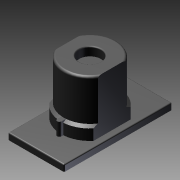
# Autodesk Inventor part: M2T12A5bush
Saved by Autodesk Inventor 2011 SP1 (Build 150282100, 282)
## iProperties
Created: 2013-12-24
Part Number: M2T12A5bush
Catalog Web Link: www.cadenas.de
Description: M2T Series - Process Sealed Miniature Toggles - Bushing-
Vendor: NKKSWITCHES
Document SubType Name: Modeling
Designer: PARTuser1
Manufacturer: NKKSWITCHES
Density: 1 g/cm^3
Category: PARTsolutions
Company: NKKSWITCHES
Title: M2T12A5bush
Author: Cadenas PARTsolutions
PSOL_IDENT_0: {$CADENAS_DATA\23d-libs\nkkswitches\toggle\m2t\parts\m2t_bushing.prj},222 {VTYP=3D},{NB=M2T12A5bush}
PSOL_IDENT_1: ,{LINA=M2T12A5bush},{NN=M2T Series - Process Sealed Miniature Toggles - Bushing},{DATE=07.04.2009 11
PSOL_IDENT_2: :51:13},{GEOMDATE=07.04.2009 11:51:00},{VERSION=},{LINEID=10},{LINESUBID=-1},{WBVAR=PLS,CRCTS}  {NB=
PSOL_IDENT_3: M2T12A5bush},{LINA=M2T12A5bush},{KT=DUMMY},{PN=M2T12A5},{SRS=M2T},{PLS=1},{CRCTS=2},{BSHNG=A5 - .250
PSOL_IDENT_4: \" (6.35mm) Double Flatted}
CNS_NN: M2T Series - Process Sealed Miniature Toggles - Bushing
CNS_NB: M2T12A5bush
CNS_NBSYN: $PN.bush
CNS_LINA: M2T12A5bush
CNS_PN: M2T12A5
CNS_SRS: M2T
CNS_PLS: 1 - SPDT
CNS_CRCTS: 2 - ON/NONE/ON
CNS_BSHNG: A5 - .250" (6.35mm) Double Flatted
SUPPLIER: NKKSWITCHES
ARTICLENO: M2T12A5bush
BOMINFO: M2T12A5bush
CREATOR: CADENAS GmbH
Autodesk Inventor part; units mm, degrees
sketch "Sketch_1" plane through (0, 0, 0) normal (0, 1, 0) x (-1, 0, 0)
  line L0 (3.302, -6.223) -> (3.302, 6.223)
  arc A0 (3.302, 6.223) -> (3.175, 6.35) centre (3.175, 6.223) ccw
  line L1 (3.175, 6.35) -> (-3.175, 6.35)
  arc A1 (-3.175, 6.35) -> (-3.302, 6.223) centre (-3.175, 6.223) ccw
  line L2 (-3.302, 6.223) -> (-3.302, -6.223)
  arc A2 (-3.302, -6.223) -> (-3.175, -6.35) centre (-3.175, -6.223) ccw
  line L3 (-3.175, -6.35) -> (3.175, -6.35)
  arc A3 (3.175, -6.35) -> (3.302, -6.223) centre (3.175, -6.223) ccw
  constraints: 8 end point, 8 point on circle, 4 centre point
extrude "Extrusion1" add sketch "Sketch_1" against normal blind 0.762
sketch "Sketch_2" plane through (0, 0, 0) normal (0, 0, 1) x (1, 0, 0)
  line L0 (-3.302, 0.254) -> (-3.302, -0.127)
  arc A0 (-3.175, 0) -> (-3.302, -0.127) centre (-3.175, -0.127) ccw
  line L1 (-3.175, 0) -> (3.175, 0)
  arc A1 (3.302, -0.127) -> (3.175, 0) centre (3.175, -0.127) ccw
  line L2 (3.302, -0.127) -> (3.302, 0.254)
  line L3 (3.302, 0.254) -> (-3.302, 0.254)
  constraints: 8 end point, 4 point on circle, 2 centre point
extrude "Extrusion2" cut sketch "Sketch_2" along normal mid plane 12.7
sketch "Sketch_3" plane through (0, 0, 0) normal (1, 0, 0) x (0, 1, 0)
  line L0 (0.254, 6.35) -> (-0.127, 6.35)
  arc A0 (0, 6.223) -> (-0.127, 6.35) centre (-0.127, 6.223) ccw
  line L1 (0, 6.223) -> (0, -6.223)
  arc A1 (-0.127, -6.35) -> (0, -6.223) centre (-0.127, -6.223) ccw
  line L2 (-0.127, -6.35) -> (0.254, -6.35)
  line L3 (0.254, -6.35) -> (0.254, 6.35)
  constraints: 8 end point, 4 point on circle, 2 centre point
extrude "Extrusion3" cut sketch "Sketch_3" along normal mid plane 12.7
sketch "Sketch_4" plane through (0, 0, 0) normal (1, 0, 0) x (0, 1, 0)
  line L0 (0, 0) -> (6.35, 0)
  line L1 (5.334, 0) -> (5.334, -1.27)
  line L2 (5.334, -1.27) -> (6.223, -1.27)
  arc A0 (6.35, -1.397) -> (6.223, -1.27) centre (6.223, -1.397) ccw
  line L3 (6.35, -1.397) -> (6.35, -2.8448)
  arc A1 (6.096, -3.0988) -> (6.35, -2.8448) centre (6.096, -2.8448) ccw
  line L4 (6.096, -3.0988) -> (1.524, -3.0988)
  line L5 (1.524, -3.0988) -> (1.27, -3.4036)
  line L6 (1.27, -3.4036) -> (0, -3.4036)
  line L7 (0, -3.4036) -> (0, 0)
  line L8 (0, 0) -> (5.334, 0)
  constraints: 18 end point, 4 point on circle, 2 centre point
revolve "Revolution1" add sketch "Sketch_4" angle 360 about axis through (0, 0, 0) along (0, -1, 0)
sketch "Sketch_5" plane through (0, 0, 0) normal (0, 1, 0) x (-1, 0, 0)
  line L0 (0.254, -3.6068) -> (0.254, 3.6068)
  arc A0 (0.254, 3.6068) -> (-0.254, 3.6068) centre (0, 3.6068) ccw
  line L1 (-0.254, 3.6068) -> (-0.254, -3.6068)
  arc A1 (-0.254, -3.6068) -> (0.254, -3.6068) centre (0, -3.6068) ccw
  constraints: 4 end point, 4 point on circle, 2 centre point
extrude "Extrusion4" add sketch "Sketch_5" along normal blind 1.524
sketch "Sketch_6" plane through (0, 6.35, 0) normal (0, 1, 0) x (1, 0, 0)
  line L0 (-3.8735, -5.08) -> (3.8735, -5.08)
  line L1 (3.8735, -5.08) -> (3.8735, 5.08)
  line L2 (3.8735, 5.08) -> (-3.8735, 5.08)
  line L3 (-3.8735, 5.08) -> (-3.8735, -5.08)
  line L4 (-2.6035, 4.572) -> (-2.6035, -4.572)
  line L5 (-2.6035, -4.572) -> (2.6035, -4.572)
  line L6 (2.6035, -4.572) -> (2.6035, 4.572)
  line L7 (2.6035, 4.572) -> (-2.6035, 4.572)
  constraints: 16 end point
extrude "Extrusion5" cut sketch "Sketch_6" against normal blind 6.35
ref_plane "body_XY" through (0, -0.762, 0) normal (0, 1, 0) x (1, 0, 0)
ref_plane "body_YZ" through (0, -0.762, 0) normal (1, 0, 0) x (0, 0, -1)
ref_plane "body_ZX" through (0, -0.762, 0) normal (0, 0, -1) x (0, 1, 0)
ref_plane "bus_brac_XY" through (0, 0, 0) normal (0, -1, 0) x (1, 0, 0)
ref_plane "bus_brac_YZ" through (0, 0, 0) normal (1, 0, 0) x (0, 0, 1)
ref_plane "bus_brac_ZX" through (0, 0, 0) normal (0, 0, 1) x (0, -1, 0)
ref_plane "toggle_XY" through (0, 6.35, 0) normal (0, -1, 0) x (1, 0, 0)
ref_plane "toggle_YZ" through (0, 6.35, 0) normal (1, 0, 0) x (0, 0, 1)
ref_plane "toggle_ZX" through (0, 6.35, 0) normal (0, 0, 1) x (0, -1, 0)
body "Solid1"
